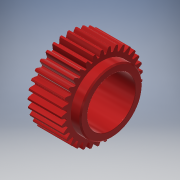
# Autodesk Inventor part: Component 20 (Planet Wheel)
Saved by Autodesk Inventor 2018 (Build 220112000, 112)
## iProperties
Created: 2023-03-16
Part Number: Component 20 (Planet Wheel)
Material: Generic
Document SubType Name: Modeling
Designer: Habib Mohamed
Density: 1 g/cm^3
Appearance: Light Red
Author: Habib Mohamed
Autodesk Inventor part; units mm, degrees
ref_plane "YZ Plane" through (0, 0, 0) normal (1, 0, 0) x (0, 1, 0)
ref_plane "XZ Plane" through (0, 0, 0) normal (0, 1, 0) x (-1, 0, 0)
ref_plane "XY Plane" through (0, 0, 0) normal (0, 0, 1) x (1, 0, 0)
sketch "Sketch1" plane through (0, 0, 0) normal (1, 0, 0) x (0, 1, 0)
  circle A0 centre (0, 0) radius 5
  circle A1 centre (0, 0) radius 6.5
  arc A2 (8.489, -0.1315) -> (8.489, 0.1315) centre (0, 0) ccw
  arc A3 (8.4261, 0.2228) -> (7.4269, 0.5117) centre (6.4759, -4.6515) ccw
  arc A4 (8.489, 0.1315) -> (8.4261, 0.2228) centre (8.389, 0.13) ccw
  arc A5 (7.3454, 0.6018) -> (7.4269, 0.5117) centre (7.4451, 0.61) ccw
  line L0 (0, 0) -> (12.5329, 0) construction
  arc A6 (7.4269, -0.5117) -> (8.4261, -0.2228) centre (6.4759, 4.6515) ccw
  arc A7 (8.4261, -0.2228) -> (8.489, -0.1315) centre (8.389, -0.13) ccw
  arc A8 (7.4269, -0.5117) -> (7.3454, -0.6018) centre (7.4451, -0.61) ccw
  arc A9 (7.0987, 1.9811) -> (7.1959, 1.908) centre (7.1951, 2.008) ccw
  arc A10 (8.3107, 1.7357) -> (8.2317, 1.8135) centre (8.2128, 1.7153) ccw
  arc A11 (8.3605, 1.4774) -> (8.3107, 1.7357) centre (0, 0) ccw
  arc A12 (7.3896, 0.9031) -> (8.316, 1.3758) centre (5.4786, 5.793) ccw
  arc A13 (7.3896, 0.9031) -> (7.3265, 0.7992) centre (7.426, 0.81) ccw
  arc A14 (8.316, 1.3758) -> (8.3605, 1.4774) centre (8.262, 1.46) ccw
  arc A15 (8.2317, 1.8135) -> (7.1959, 1.908) centre (7.2392, -3.3419) ccw
  arc A16 (6.5955, 3.2887) -> (6.7048, 3.2353) centre (6.685, 3.3334) ccw
  arc A17 (7.832, 3.2772) -> (7.7397, 3.3386) centre (7.7398, 3.2386) ccw
  arc A18 (7.9298, 3.0329) -> (7.832, 3.2772) centre (0, 0) ccw
  arc A19 (7.0851, 2.2853) -> (7.9054, 2.9248) centre (4.2833, 6.7252) ccw
  arc A20 (7.0851, 2.2853) -> (7.0429, 2.1713) centre (7.1385, 2.2007) ccw
  arc A21 (7.9054, 2.9248) -> (7.9298, 3.0329) centre (7.8364, 2.9972) ccw
  arc A22 (7.7397, 3.3386) -> (6.7048, 3.2353) centre (7.7408, -1.9114) ccw
  arc A23 (5.854, 4.4775) -> (5.9713, 4.4457) centre (5.9334, 4.5383) ccw
  arc A24 (7.0703, 4.7002) -> (6.968, 4.743) centre (6.987, 4.6448) ccw
  arc A25 (7.2125, 4.4788) -> (7.0703, 4.7002) centre (0, 0) ccw
  arc A26 (6.5246, 3.5849) -> (7.209, 4.368) centre (2.9331, 7.4142) ccw
  arc A27 (6.5246, 3.5849) -> (6.5047, 3.4649) centre (6.593, 3.5119) ccw
  arc A28 (7.209, 4.368) -> (7.2125, 4.4788) centre (7.1276, 4.4261) ccw
  arc A29 (6.968, 4.743) -> (5.9713, 4.4457) centre (7.9627, -0.4119) ccw
  arc A30 (4.9008, 5.5045) -> (5.022, 5.4955) centre (4.9673, 5.5792) ccw
  arc A31 (6.053, 5.9533) -> (5.9445, 5.976) centre (5.9817, 5.8832) ccw
  arc A32 (6.2345, 5.7629) -> (6.053, 5.9533) centre (0, 0) ccw
  arc A33 (5.7282, 4.7549) -> (6.2521, 5.6534) centre (1.4769, 7.8353) ccw
  arc A34 (5.7282, 4.7549) -> (5.7314, 4.6333) centre (5.8092, 4.6962) ccw
  arc A35 (6.2521, 5.6534) -> (6.2345, 5.7629) centre (6.1611, 5.695) ccw
  arc A36 (5.9445, 5.976) -> (5.022, 5.4955) centre (7.8967, 1.1025) ccw
  arc A37 (3.7705, 6.3325) -> (3.8913, 6.3466) centre (3.8217, 6.4184) ccw
  arc A38 (4.8169, 6.9912) -> (4.7061, 6.993) centre (4.7602, 6.9089) ccw
  arc A39 (5.0312, 6.8386) -> (4.8169, 6.9912) centre (0, 0) ccw
  arc A40 (4.7248, 5.753) -> (5.0692, 6.7345) centre (-0.0326, 7.9733) ccw
  arc A41 (4.7248, 5.753) -> (4.751, 5.6343) centre (4.8154, 5.7107) ccw
  arc A42 (5.0692, 6.7345) -> (5.0312, 6.8386) centre (4.972, 6.7581) ccw
  arc A43 (4.7061, 6.993) -> (3.8913, 6.3466) centre (7.5454, 2.577) ccw
  arc A44 (2.5039, 6.9316) -> (2.6198, 6.9683) centre (2.5379, 7.0257) ccw
  arc A45 (3.4068, 7.7765) -> (3.2976, 7.7573) centre (3.3667, 7.6849) ccw
  arc A46 (3.6461, 7.6672) -> (3.4068, 7.7765) centre (0, 0) ccw
  arc A47 (3.5507, 6.5432) -> (3.7031, 7.5721) centre (-1.541, 7.823) ccw
  arc A48 (3.5507, 6.5432) -> (3.5988, 6.4316) centre (3.6477, 6.5189) ccw
  arc A49 (3.7031, 7.5721) -> (3.6461, 7.6672) centre (3.6032, 7.5769) ccw
  arc A50 (3.2976, 7.7573) -> (2.6198, 6.9683) centre (6.9213, 3.9584) ccw
  arc A51 (1.1469, 7.2802) -> (1.2537, 7.3382) centre (1.1624, 7.379) ccw
  arc A52 (1.8735, 8.2807) -> (1.77, 8.2412) centre (1.8514, 8.1832) ccw
  arc A53 (2.1292, 8.2187) -> (1.8735, 8.2807) centre (0, 0) ccw
  arc A54 (2.2482, 7.097) -> (2.2031, 8.1361) centre (-2.9936, 7.39) ccw
  arc A55 (2.2482, 7.097) -> (2.3166, 6.9964) centre (2.348, 7.0914) ccw
  arc A56 (2.2031, 8.1361) -> (2.1292, 8.2187) centre (2.1041, 8.1219) ccw
  arc A57 (1.77, 8.2412) -> (1.2537, 7.3382) centre (6.0471, 5.1967) ccw
  arc A58 (-0.2516, 7.3657) -> (-0.1577, 7.4429) centre (-0.2551, 7.4656) ccw
  arc A59 (0.2725, 8.4856) -> (0.1783, 8.4272) centre (0.2693, 8.3857) ccw
  arc A60 (0.5353, 8.4731) -> (0.2725, 8.4856) centre (0, 0) ccw
  arc A61 (0.8645, 7.3942) -> (0.6235, 8.406) centre (-4.3381, 6.6899) ccw
  arc A62 (0.8645, 7.3942) -> (0.9507, 7.3084) centre (0.9636, 7.4076) ccw
  arc A63 (0.6235, 8.406) -> (0.5353, 8.4731) centre (0.529, 8.3733) ccw
  arc A64 (0.1783, 8.4272) -> (-0.1577, 7.4429) centre (4.9544, 6.2473) ccw
  arc A65 (-1.6411, 7.185) -> (-1.5634, 7.2785) centre (-1.6633, 7.2825) ccw
  arc A66 (-1.3383, 8.3839) -> (-1.4197, 8.3087) centre (-1.3226, 8.2851) ccw
  arc A67 (-1.0779, 8.4213) -> (-1.3383, 8.3839) centre (0, 0) ccw
  arc A68 (-0.5505, 7.4242) -> (-0.9786, 8.3721) centre (-5.5258, 5.748) ccw
  arc A69 (-0.5505, 7.4242) -> (-0.4496, 7.3563) centre (-0.4558, 7.4561) ccw
  arc A70 (-0.9786, 8.3721) -> (-1.0779, 8.4213) centre (-1.0652, 8.3221) ccw
  arc A71 (-1.4197, 8.3087) -> (-1.5634, 7.2785) centre (3.6825, 7.072) ccw
  arc A72 (-2.9712, 6.7446) -> (-2.9126, 6.8511) centre (-3.0115, 6.8361) ccw
  arc A73 (-2.9008, 7.9791) -> (-2.9665, 7.8898) centre (-2.8666, 7.8851) ccw
  arc A74 (-2.6522, 8.0651) -> (-2.9008, 7.9791) centre (0, 0) ccw
  arc A75 (-1.9456, 7.1858) -> (-2.5453, 8.0356) centre (-6.5137, 4.5984) ccw
  arc A76 (-1.9456, 7.1858) -> (-1.8337, 7.1382) centre (-1.8586, 7.2351) ccw
  arc A77 (-2.5453, 8.0356) -> (-2.6522, 8.0651) centre (-2.6209, 7.9701) ccw
  arc A78 (-2.9665, 7.8898) -> (-2.9126, 6.8511) centre (2.2776, 7.6411) ccw
  arc A79 (-4.1939, 6.0604) -> (-4.1566, 6.1761) centre (-4.2508, 6.1426) ccw
  arc A80 (-4.3584, 7.2859) -> (-4.4061, 7.1858) centre (-4.3071, 7.2001) ccw
  arc A81 (-4.1306, 7.4174) -> (-4.3584, 7.2859) centre (0, 0) ccw
  arc A82 (-3.2704, 6.6877) -> (-4.0201, 7.4087) centre (-7.2663, 3.2826) ccw
  arc A83 (-3.2704, 6.6877) -> (-3.1515, 6.6622) centre (-3.1943, 6.7526) ccw
  arc A84 (-4.0201, 7.4087) -> (-4.1306, 7.4174) centre (-4.0819, 7.3301) ccw
  arc A85 (-4.4061, 7.1858) -> (-4.1566, 6.1761) centre (0.7903, 7.9341) ccw
  arc A86 (-5.265, 5.1572) -> (-5.2503, 5.2778) centre (-5.3365, 5.2271) ccw
  arc A87 (-5.6585, 6.3294) -> (-5.6864, 6.2221) centre (-5.5919, 6.2548) ccw
  arc A88 (-5.4597, 6.5017) -> (-5.6585, 6.3294) centre (0, 0) ccw
  arc A89 (-4.4769, 5.948) -> (-5.3495, 6.514) centre (-7.7562, 1.8481) ccw
  arc A90 (-4.4769, 5.948) -> (-4.3554, 5.9454) centre (-4.4145, 6.0261) ccw
  arc A91 (-5.3495, 6.514) -> (-5.4597, 6.5017) centre (-5.3954, 6.4251) ccw
  arc A92 (-5.6864, 6.2221) -> (-5.2503, 5.2778) centre (-0.7255, 7.9403) ccw
  arc A93 (-6.1459, 4.0675) -> (-6.1543, 4.1888) centre (-6.2293, 4.1227) ccw
  arc A94 (-6.7541, 5.1441) -> (-6.7611, 5.0335) centre (-6.6746, 5.0835) ccw
  arc A95 (-6.5915, 5.3509) -> (-6.7541, 5.1441) centre (0, 0) ccw
  arc A96 (-5.5217, 4.9932) -> (-6.4856, 5.3839) centre (-7.9658, 0.3468) ccw
  arc A97 (-5.5217, 4.9932) -> (-5.4018, 5.0137) centre (-5.4751, 5.0817) ccw
  arc A98 (-6.4856, 5.3839) -> (-6.5915, 5.3509) centre (-6.5138, 5.2879) ccw
  arc A99 (-6.7611, 5.0335) -> (-6.1543, 4.1888) centre (-2.2151, 7.6595) ccw
  arc A100 (-6.8046, 2.8309) -> (-6.8358, 2.9484) centre (-6.8969, 2.8693) ccw
  arc A101 (-7.6056, 3.773) -> (-7.5916, 3.663) centre (-7.516, 3.7285) ccw
  arc A102 (-7.485, 4.0068) -> (-7.6056, 3.773) centre (0, 0) ccw
  arc A103 (-6.3669, 3.858) -> (-7.3873, 4.0592) centre (-7.8875, -1.167) ccw
  arc A104 (-6.3669, 3.858) -> (-6.2531, 3.9008) centre (-6.3379, 3.9537) ccw
  arc A105 (-7.3873, 4.0592) -> (-7.485, 4.0068) centre (-7.3969, 3.9596) ccw
  arc A106 (-7.5916, 3.663) -> (-6.8358, 2.9484) centre (-3.6246, 7.1018) ccw
  arc A107 (-7.2174, 1.492) -> (-7.2702, 1.6015) centre (-7.3153, 1.5122) ccw
  arc A108 (-8.1822, 2.2654) -> (-8.1476, 2.1601) centre (-8.0858, 2.2387) ccw
  arc A109 (-8.1081, 2.5178) -> (-8.1822, 2.2654) centre (0, 0) ccw
  arc A110 (-6.9819, 2.5833) -> (-8.022, 2.5877) centre (-7.5241, -2.6386) ccw
  arc A111 (-6.9819, 2.5833) -> (-6.8783, 2.6469) centre (-6.9716, 2.6828) ccw
  arc A112 (-8.022, 2.5877) -> (-8.1081, 2.5178) centre (-8.0126, 2.4882) ccw
  arc A113 (-8.1476, 2.1601) -> (-7.2702, 1.6015) centre (-4.9031, 6.2875) ccw
  arc A114 (-7.3693, 0.0991) -> (-7.4419, 0.1966) centre (-7.4693, 0.1005) ccw
  arc A115 (-8.463, 0.676) -> (-8.4092, 0.5791) centre (-8.3634, 0.668) ccw
  arc A116 (-8.438, 0.9379) -> (-8.463, 0.676) centre (0, 0) ccw
  arc A117 (-7.3447, 1.2153) -> (-8.3668, 1.0228) centre (-6.8887, -4.0149) ccw
  arc A118 (-7.3447, 1.2153) -> (-7.2549, 1.2973) centre (-7.3534, 1.3149) ccw
  arc A119 (-8.3668, 1.0228) -> (-8.438, 0.9379) centre (-8.3386, 0.9268) ccw
  arc A120 (-8.4092, 0.5791) -> (-7.4419, 0.1966) centre (-6.0044, 5.246) ccw
  arc A121 (-7.2549, -1.2973) -> (-7.3447, -1.2153) centre (-7.3534, -1.3149) ccw
  arc A122 (-8.438, -0.9379) -> (-8.3668, -1.0228) centre (-8.3386, -0.9268) ccw
  arc A123 (-8.463, -0.676) -> (-8.438, -0.9379) centre (0, 0) ccw
  arc A124 (-7.4419, -0.1966) -> (-8.4092, -0.5791) centre (-6.0044, -5.246) ccw
  arc A125 (-7.4419, -0.1966) -> (-7.3693, -0.0991) centre (-7.4693, -0.1005) ccw
  arc A126 (-8.4092, -0.5791) -> (-8.463, -0.676) centre (-8.3634, -0.668) ccw
  arc A127 (-8.3668, -1.0228) -> (-7.3447, -1.2153) centre (-6.8887, 4.0149) ccw
  arc A128 (-6.8783, -2.6469) -> (-6.9819, -2.5833) centre (-6.9716, -2.6828) ccw
  arc A129 (-8.1081, -2.5178) -> (-8.022, -2.5877) centre (-8.0126, -2.4882) ccw
  arc A130 (-8.1822, -2.2654) -> (-8.1081, -2.5178) centre (0, 0) ccw
  arc A131 (-7.2702, -1.6015) -> (-8.1476, -2.1601) centre (-4.9031, -6.2875) ccw
  arc A132 (-7.2702, -1.6015) -> (-7.2174, -1.492) centre (-7.3153, -1.5122) ccw
  arc A133 (-8.1476, -2.1601) -> (-8.1822, -2.2654) centre (-8.0858, -2.2387) ccw
  arc A134 (-8.022, -2.5877) -> (-6.9819, -2.5833) centre (-7.5241, 2.6386) ccw
  arc A135 (-6.2531, -3.9008) -> (-6.3669, -3.858) centre (-6.3379, -3.9537) ccw
  arc A136 (-7.485, -4.0068) -> (-7.3873, -4.0592) centre (-7.3969, -3.9596) ccw
  arc A137 (-7.6056, -3.773) -> (-7.485, -4.0068) centre (0, 0) ccw
  arc A138 (-6.8358, -2.9484) -> (-7.5916, -3.663) centre (-3.6246, -7.1018) ccw
  arc A139 (-6.8358, -2.9484) -> (-6.8046, -2.8309) centre (-6.8969, -2.8693) ccw
  arc A140 (-7.5916, -3.663) -> (-7.6056, -3.773) centre (-7.516, -3.7285) ccw
  arc A141 (-7.3873, -4.0592) -> (-6.3669, -3.858) centre (-7.8875, 1.167) ccw
  arc A142 (-5.4018, -5.0137) -> (-5.5217, -4.9932) centre (-5.4751, -5.0817) ccw
  arc A143 (-6.5915, -5.3509) -> (-6.4856, -5.3839) centre (-6.5138, -5.2879) ccw
  arc A144 (-6.7541, -5.1441) -> (-6.5915, -5.3509) centre (0, 0) ccw
  arc A145 (-6.1543, -4.1888) -> (-6.7611, -5.0335) centre (-2.2151, -7.6595) ccw
  arc A146 (-6.1543, -4.1888) -> (-6.1459, -4.0675) centre (-6.2293, -4.1227) ccw
  arc A147 (-6.7611, -5.0335) -> (-6.7541, -5.1441) centre (-6.6746, -5.0835) ccw
  arc A148 (-6.4856, -5.3839) -> (-5.5217, -4.9932) centre (-7.9658, -0.3468) ccw
  arc A149 (-4.3554, -5.9454) -> (-4.4769, -5.948) centre (-4.4145, -6.0261) ccw
  arc A150 (-5.4597, -6.5017) -> (-5.3495, -6.514) centre (-5.3954, -6.4251) ccw
  arc A151 (-5.6585, -6.3294) -> (-5.4597, -6.5017) centre (0, 0) ccw
  arc A152 (-5.2503, -5.2778) -> (-5.6864, -6.2221) centre (-0.7255, -7.9403) ccw
  arc A153 (-5.2503, -5.2778) -> (-5.265, -5.1572) centre (-5.3365, -5.2271) ccw
  arc A154 (-5.6864, -6.2221) -> (-5.6585, -6.3294) centre (-5.5919, -6.2548) ccw
  arc A155 (-5.3495, -6.514) -> (-4.4769, -5.948) centre (-7.7562, -1.8481) ccw
  arc A156 (-3.1515, -6.6622) -> (-3.2704, -6.6877) centre (-3.1943, -6.7526) ccw
  arc A157 (-4.1306, -7.4174) -> (-4.0201, -7.4087) centre (-4.0819, -7.3301) ccw
  arc A158 (-4.3584, -7.2859) -> (-4.1306, -7.4174) centre (0, 0) ccw
  arc A159 (-4.1566, -6.1761) -> (-4.4061, -7.1858) centre (0.7903, -7.9341) ccw
  arc A160 (-4.1566, -6.1761) -> (-4.1939, -6.0604) centre (-4.2508, -6.1426) ccw
  arc A161 (-4.4061, -7.1858) -> (-4.3584, -7.2859) centre (-4.3071, -7.2001) ccw
  arc A162 (-4.0201, -7.4087) -> (-3.2704, -6.6877) centre (-7.2663, -3.2826) ccw
  arc A163 (-1.8337, -7.1382) -> (-1.9456, -7.1858) centre (-1.8586, -7.2351) ccw
  arc A164 (-2.6522, -8.0651) -> (-2.5453, -8.0356) centre (-2.6209, -7.9701) ccw
  arc A165 (-2.9008, -7.9791) -> (-2.6522, -8.0651) centre (0, 0) ccw
  arc A166 (-2.9126, -6.8511) -> (-2.9665, -7.8898) centre (2.2776, -7.6411) ccw
  arc A167 (-2.9126, -6.8511) -> (-2.9712, -6.7446) centre (-3.0115, -6.8361) ccw
  arc A168 (-2.9665, -7.8898) -> (-2.9008, -7.9791) centre (-2.8666, -7.8851) ccw
  arc A169 (-2.5453, -8.0356) -> (-1.9456, -7.1858) centre (-6.5137, -4.5984) ccw
  arc A170 (-0.4496, -7.3563) -> (-0.5505, -7.4242) centre (-0.4558, -7.4561) ccw
  arc A171 (-1.0779, -8.4213) -> (-0.9786, -8.3721) centre (-1.0652, -8.3221) ccw
  arc A172 (-1.3383, -8.3839) -> (-1.0779, -8.4213) centre (0, 0) ccw
  arc A173 (-1.5634, -7.2785) -> (-1.4197, -8.3087) centre (3.6825, -7.072) ccw
  arc A174 (-1.5634, -7.2785) -> (-1.6411, -7.185) centre (-1.6633, -7.2825) ccw
  arc A175 (-1.4197, -8.3087) -> (-1.3383, -8.3839) centre (-1.3226, -8.2851) ccw
  arc A176 (-0.9786, -8.3721) -> (-0.5505, -7.4242) centre (-5.5258, -5.748) ccw
  arc A177 (0.9507, -7.3084) -> (0.8645, -7.3942) centre (0.9636, -7.4076) ccw
  arc A178 (0.5353, -8.4731) -> (0.6235, -8.406) centre (0.529, -8.3733) ccw
  arc A179 (0.2725, -8.4856) -> (0.5353, -8.4731) centre (0, 0) ccw
  arc A180 (-0.1577, -7.4429) -> (0.1783, -8.4272) centre (4.9544, -6.2473) ccw
  arc A181 (-0.1577, -7.4429) -> (-0.2516, -7.3657) centre (-0.2551, -7.4656) ccw
  arc A182 (0.1783, -8.4272) -> (0.2725, -8.4856) centre (0.2693, -8.3857) ccw
  arc A183 (0.6235, -8.406) -> (0.8645, -7.3942) centre (-4.3381, -6.6899) ccw
  arc A184 (2.3166, -6.9964) -> (2.2482, -7.097) centre (2.348, -7.0914) ccw
  arc A185 (2.1292, -8.2187) -> (2.2031, -8.1361) centre (2.1041, -8.1219) ccw
  arc A186 (1.8735, -8.2807) -> (2.1292, -8.2187) centre (0, 0) ccw
  arc A187 (1.2537, -7.3382) -> (1.77, -8.2412) centre (6.0471, -5.1967) ccw
  arc A188 (1.2537, -7.3382) -> (1.1469, -7.2802) centre (1.1624, -7.379) ccw
  arc A189 (1.77, -8.2412) -> (1.8735, -8.2807) centre (1.8514, -8.1832) ccw
  arc A190 (2.2031, -8.1361) -> (2.2482, -7.097) centre (-2.9936, -7.39) ccw
  arc A191 (3.5988, -6.4316) -> (3.5507, -6.5432) centre (3.6477, -6.5189) ccw
  arc A192 (3.6461, -7.6672) -> (3.7031, -7.5721) centre (3.6032, -7.5769) ccw
  arc A193 (3.4068, -7.7765) -> (3.6461, -7.6672) centre (0, 0) ccw
  arc A194 (2.6198, -6.9683) -> (3.2976, -7.7573) centre (6.9213, -3.9584) ccw
  arc A195 (2.6198, -6.9683) -> (2.5039, -6.9316) centre (2.5379, -7.0257) ccw
  arc A196 (3.2976, -7.7573) -> (3.4068, -7.7765) centre (3.3667, -7.6849) ccw
  arc A197 (3.7031, -7.5721) -> (3.5507, -6.5432) centre (-1.541, -7.823) ccw
  arc A198 (4.751, -5.6343) -> (4.7248, -5.753) centre (4.8154, -5.7107) ccw
  arc A199 (5.0312, -6.8386) -> (5.0692, -6.7345) centre (4.972, -6.7581) ccw
  arc A200 (4.8169, -6.9912) -> (5.0312, -6.8386) centre (0, 0) ccw
  arc A201 (3.8913, -6.3466) -> (4.7061, -6.993) centre (7.5454, -2.577) ccw
  arc A202 (3.8913, -6.3466) -> (3.7705, -6.3325) centre (3.8217, -6.4184) ccw
  arc A203 (4.7061, -6.993) -> (4.8169, -6.9912) centre (4.7602, -6.9089) ccw
  arc A204 (5.0692, -6.7345) -> (4.7248, -5.753) centre (-0.0326, -7.9733) ccw
  arc A205 (5.7314, -4.6333) -> (5.7282, -4.7549) centre (5.8092, -4.6962) ccw
  arc A206 (6.2345, -5.7629) -> (6.2521, -5.6534) centre (6.1611, -5.695) ccw
  arc A207 (6.053, -5.9533) -> (6.2345, -5.7629) centre (0, 0) ccw
  arc A208 (5.022, -5.4955) -> (5.9445, -5.976) centre (7.8967, -1.1025) ccw
  arc A209 (5.022, -5.4955) -> (4.9008, -5.5045) centre (4.9673, -5.5792) ccw
  arc A210 (5.9445, -5.976) -> (6.053, -5.9533) centre (5.9817, -5.8832) ccw
  arc A211 (6.2521, -5.6534) -> (5.7282, -4.7549) centre (1.4769, -7.8353) ccw
  arc A212 (6.5047, -3.4649) -> (6.5246, -3.5849) centre (6.593, -3.5119) ccw
  arc A213 (7.2125, -4.4788) -> (7.209, -4.368) centre (7.1276, -4.4261) ccw
  arc A214 (7.0703, -4.7002) -> (7.2125, -4.4788) centre (0, 0) ccw
  arc A215 (5.9713, -4.4457) -> (6.968, -4.743) centre (7.9627, 0.4119) ccw
  arc A216 (5.9713, -4.4457) -> (5.854, -4.4775) centre (5.9334, -4.5383) ccw
  arc A217 (6.968, -4.743) -> (7.0703, -4.7002) centre (6.987, -4.6448) ccw
  arc A218 (7.209, -4.368) -> (6.5246, -3.5849) centre (2.9331, -7.4142) ccw
  arc A219 (7.0429, -2.1713) -> (7.0851, -2.2853) centre (7.1385, -2.2007) ccw
  arc A220 (7.9298, -3.0329) -> (7.9054, -2.9248) centre (7.8364, -2.9972) ccw
  arc A221 (7.832, -3.2772) -> (7.9298, -3.0329) centre (0, 0) ccw
  arc A222 (6.7048, -3.2353) -> (7.7397, -3.3386) centre (7.7408, 1.9114) ccw
  arc A223 (6.7048, -3.2353) -> (6.5955, -3.2887) centre (6.685, -3.3334) ccw
  arc A224 (7.7397, -3.3386) -> (7.832, -3.2772) centre (7.7398, -3.2386) ccw
  arc A225 (7.9054, -2.9248) -> (7.0851, -2.2853) centre (4.2833, -6.7252) ccw
  arc A226 (7.3265, -0.7992) -> (7.3896, -0.9031) centre (7.426, -0.81) ccw
  arc A227 (8.3605, -1.4774) -> (8.316, -1.3758) centre (8.262, -1.46) ccw
  arc A228 (8.3107, -1.7357) -> (8.3605, -1.4774) centre (0, 0) ccw
  arc A229 (7.1959, -1.908) -> (8.2317, -1.8135) centre (7.2392, 3.3419) ccw
  arc A230 (7.1959, -1.908) -> (7.0987, -1.9811) centre (7.1951, -2.008) ccw
  arc A231 (8.2317, -1.8135) -> (8.3107, -1.7357) centre (8.2128, -1.7153) ccw
  arc A232 (8.316, -1.3758) -> (7.3896, -0.9031) centre (5.4786, -5.793) ccw
  arc A233 (7.0987, 1.9811) -> (7.0429, 2.1713) centre (0, 0) ccw
  arc A234 (7.3454, 0.6018) -> (7.3265, 0.7992) centre (0, 0) ccw
  arc A235 (7.3265, -0.7992) -> (7.3454, -0.6018) centre (0, 0) ccw
  arc A236 (6.5955, 3.2887) -> (6.5047, 3.4649) centre (0, 0) ccw
  arc A237 (5.854, 4.4775) -> (5.7314, 4.6333) centre (0, 0) ccw
  arc A238 (4.9008, 5.5045) -> (4.751, 5.6343) centre (0, 0) ccw
  arc A239 (3.7705, 6.3325) -> (3.5988, 6.4316) centre (0, 0) ccw
  arc A240 (2.5039, 6.9316) -> (2.3166, 6.9964) centre (0, 0) ccw
  arc A241 (1.1469, 7.2802) -> (0.9507, 7.3084) centre (0, 0) ccw
  arc A242 (-0.2516, 7.3657) -> (-0.4496, 7.3563) centre (0, 0) ccw
  arc A243 (-1.6411, 7.185) -> (-1.8337, 7.1382) centre (0, 0) ccw
  arc A244 (-2.9712, 6.7446) -> (-3.1515, 6.6622) centre (0, 0) ccw
  arc A245 (-4.1939, 6.0604) -> (-4.3554, 5.9454) centre (0, 0) ccw
  arc A246 (-5.265, 5.1572) -> (-5.4018, 5.0137) centre (0, 0) ccw
  arc A247 (-6.1459, 4.0675) -> (-6.2531, 3.9008) centre (0, 0) ccw
  arc A248 (-6.8046, 2.8309) -> (-6.8783, 2.6469) centre (0, 0) ccw
  arc A249 (-7.2174, 1.492) -> (-7.2549, 1.2973) centre (0, 0) ccw
  arc A250 (-7.3693, 0.0991) -> (-7.3693, -0.0991) centre (0, 0) ccw
  arc A251 (-7.2549, -1.2973) -> (-7.2174, -1.492) centre (0, 0) ccw
  arc A252 (-6.8783, -2.6469) -> (-6.8046, -2.8309) centre (0, 0) ccw
  arc A253 (-6.2531, -3.9008) -> (-6.1459, -4.0675) centre (0, 0) ccw
  arc A254 (-5.4018, -5.0137) -> (-5.265, -5.1572) centre (0, 0) ccw
  arc A255 (-4.3554, -5.9454) -> (-4.1939, -6.0604) centre (0, 0) ccw
  arc A256 (-3.1515, -6.6622) -> (-2.9712, -6.7446) centre (0, 0) ccw
  arc A257 (-1.8337, -7.1382) -> (-1.6411, -7.185) centre (0, 0) ccw
  arc A258 (-0.4496, -7.3563) -> (-0.2516, -7.3657) centre (0, 0) ccw
  arc A259 (0.9507, -7.3084) -> (1.1469, -7.2802) centre (0, 0) ccw
  arc A260 (2.3166, -6.9964) -> (2.5039, -6.9316) centre (0, 0) ccw
  arc A261 (3.5988, -6.4316) -> (3.7705, -6.3325) centre (0, 0) ccw
  arc A262 (4.751, -5.6343) -> (4.9008, -5.5045) centre (0, 0) ccw
  arc A263 (5.7314, -4.6333) -> (5.854, -4.4775) centre (0, 0) ccw
  arc A264 (6.5047, -3.4649) -> (6.5955, -3.2887) centre (0, 0) ccw
  arc A265 (7.0429, -2.1713) -> (7.0987, -1.9811) centre (0, 0) ccw
  dimension "d0" = 10
  dimension "d1" = 16.98
  dimension "d3" = 13
  dimension "d4" = 5.25
  dimension "d5" = 0.2
  dimension "d6" = 0.13
  dimension "d7" = 0.61
  dimension "d10" = 360
  constraints: 462 point on circle, 233 centre point, 7 symmetric about line, 3 tangent, 2 coincident, 2 end point, 1 equal radius, 1 horizontal, 1 vertical alignment, 830 other
  measures "d0" diameter of A0
  measures "d1" diameter of A2
  measures "d3" diameter of A1
  measures "d4" radius of A3
  measures "d5" diameter of A5
  measures "d6" distance from line of A4.centre L0
  measures "d7" distance from line of A5.centre L0
extrude "Extrusion1" add sketch "Sketch1" along normal blind 7 contours A1 | A7 A6 A8 A235 A226 A232 A227 A228 A231 A229 A230 A265 A219 A225 A220 A221 A224 A222 A223 A264 A212 A218 A213 A214 A217 A215 A216 A263 A205 A211 A206 A207 A210 A208 A209 A262 A198 A204 A199 A200 A203 A201 A202 A261 A191 A197 A192 A193 A196 A194 A195 A260 A184 A190 A185 A186 A189 A187 A188 A259 A177 A183 A178 A179 A182 A180 A181 A258 A170 A176 A171 A172 A175 A173 A174 A257 A163 A169 A164 A165 A168 A166 A167 A256 A156 A162 A157 A158 A161 A159 A160 A255 A149 A155 A150 A151 A154 A152 A153 A254 A142 A148 A143 A144 A147 A145 A146 A253 A135 A141 A136 A137 A140 A138 A139 A252 A128 A134 A129 A130 A133 A131 A132 A251 A121 A127 A122 A123 A126 A124 A125 A250 A114 A120 A115 A116 A119 A117 A118 A249 A107 A113 A108 A109 A112 A110 A111 A248 A100 A106 A101 A102 A105 A103 A104 A247 A93 A99 A94 A95 A98 A96 A97 A246 A86 A92 A87 A88 A91 A89 A90 A245 A79 A85 A80 A81 A84 A82 A83 A244 A72 A78 A73 A74 A77 A75 A76 A243 A65 A71 A66 A67 A70 A68 A69 A242 A58 A64 A59 A60 A63 A61 A62 A241 A51 A57 A52 A53 A56 A54 A55 A240 A44 A50 A45 A46 A49 A47 A48 A239 A37 A43 A38 A39 A42 A40 A41 A238 A30 A36 A31 A32 A35 A33 A34 A237 A23 A29 A24 A25 A28 A26 A27 A236 A16 A22 A17 A18 A21 A19 A20 A233 A9 A15 A10 A11 A14 A12 A13 A234 A5 A3 A4 A2
extrude "Extrusion2" add sketch "Sketch1" along normal blind 2 from surface at 7 contours A1
fillet "Fillet1" radius 0.1 2 edges at (9, -5, 0) (0, -5, 0)
chamfer "Chamfer1" distance 0.25 angle 45 1 edges at (9, -6.5, 0)
body "Solid1"
